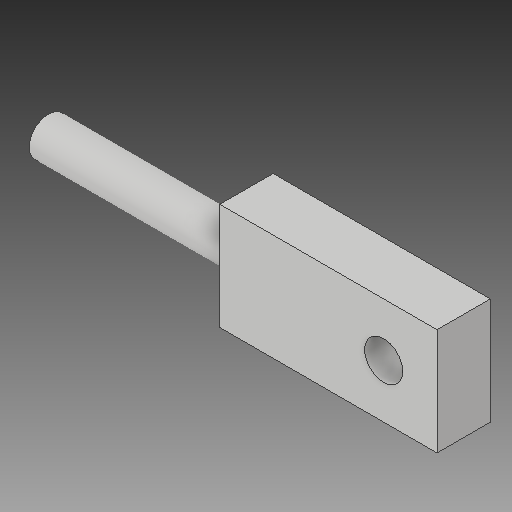
# Autodesk Inventor part: MSAL Pushing Thing
Saved by Autodesk Inventor 2019.4 (Build 234330000, 330)
## iProperties
Created: 2020-01-02
Part Number: MSAL Pushing Thing
Material: Generic
Document SubType Name: Modeling
Designer: Mark
Density: 1 g/cm^3
Appearance: Default
Author: Mark
Autodesk Inventor part; units mm, degrees
ref_plane "YZ Plane" through (0, 0, 0) normal (1, 0, 0) x (0, 1, 0)
ref_plane "XZ Plane" through (0, 0, 0) normal (0, 1, 0) x (-1, 0, 0)
ref_plane "XY Plane" through (0, 0, 0) normal (0, 0, 1) x (1, 0, 0)
sketch "Sketch1" plane through (0, 0, 0) normal (0, 0, 1) x (1, 0, 0)
  line L0 (-47.5, -14) -> (47.5, -14)
  line L1 (47.5, -14) -> (47.5, 14)
  line L2 (47.5, 14) -> (-47.5, 14)
  line L3 (-47.5, 14) -> (-47.5, -14)
  line L4 (-47.5, -14) -> (47.5, 14) construction
  line L5 (47.5, -14) -> (-47.5, 14) construction
  line L6 (47.5, 14) -> (61.5, 14)
  line L7 (61.5, 14) -> (61.5, -14)
  line L8 (61.5, -14) -> (47.5, -14)
  line L9 (47.5, -14) -> (47.5, 14)
  point P0 (0, 0)
  dimension "d0" = 95
  dimension "d1" = 28
  dimension "d2" = 14
  dimension "d3" = 28
  constraints: 20 end point, 4 parallel, 2 horizontal, 2 midpoint, 2 perpendicular
  measures "d0" distance of L2.end L1.end
  measures "d1" distance of L0.end L1.end
  measures "d2" distance of L7.end L8.end
  measures "d3" distance of L6.end L7.end
extrude "Extrusion1" add sketch "Sketch1" along normal blind 14
sketch "Sketch2" plane through (0, 0, 14) normal (0, 0, 1) x (1, 0, 0)
  circle A0 centre (47.5, 0) radius 5
  line L0 (61.5, -14) -> (61.5, 14) projected
  line L1 (-47.5, -14) -> (61.5, -14) projected
  point P0 (0, 0)
  dimension "d6" = 10
  dimension "d7" = 14
  dimension "d8" = 14
  constraints: 1 centre point
  measures "d6" diameter of A0
  measures "d7" distance from line of L0 A0.centre
  measures "d8" distance from line of L1 A0.centre
extrude "Extrusion2" cut sketch "Sketch2" against normal blind 14
sketch "Sketch3" plane through (-47.5, -14, 0) normal (-1, 0, 0) x (0, 0, 1)
  circle A0 centre (7, 14) radius 5
  line L0 (0, 28) -> (14, 28) projected
  line L1 (14, 28) -> (14, 0) projected
  circle A1 centre (7, 14) radius 25
  point P0 (0, 14)
  dimension "d11" = 10
  dimension "d12" = 14
  dimension "d13" = 7
  dimension "d14" = 50
  constraints: 2 centre point, 1 coincident
  measures "d11" diameter of A0
  measures "d12" distance from line of L0 A0.centre
  measures "d13" distance from line of L1 A0.centre
  measures "d14" diameter of A1
extrude "Extrusion3" cut sketch "Sketch3" against normal blind 52
body "Solid1"
